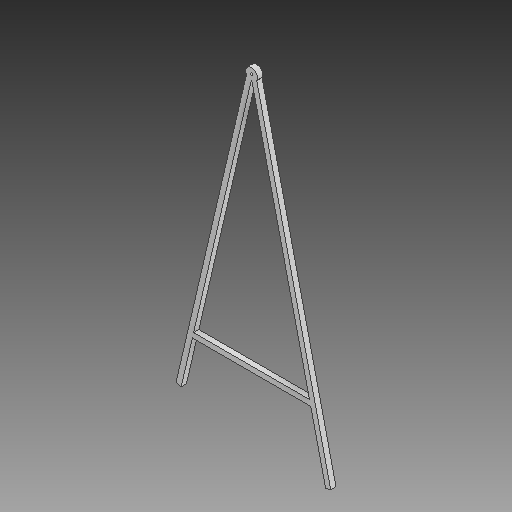
# Autodesk Inventor part: Steher
Saved by Autodesk Inventor 2021 (Build 250183000, 183)
## iProperties
Created: 2021-08-02
Part Number: Steher
Material: Generisch
Document SubType Name: Modeling
Designer: lukas
Density: 1 g/cm^3
Appearance: Vorgabe
Stock Number: Steher
Author: lukas
Autodesk Inventor part; units mm, degrees
ref_plane "YZ Plane" through (0, 0, 0) normal (1, 0, 0) x (0, 1, 0)
ref_plane "XZ Plane" through (0, 0, 0) normal (0, 1, 0) x (-1, 0, 0)
ref_plane "XY Plane" through (0, 0, 0) normal (0, 0, 1) x (1, 0, 0)
sketch "Skizze1" plane through (0, 0, 0) normal (0, 0, 1) x (1, 0, 0)
  line L0 (-523.9247, 0) -> (524.0578, 0) projected
  line L1 (0, -301.1361) -> (0, 1806.8169) projected
  line L2 (350, 0) -> (-350, 0) construction
  line L3 (-350, 0) -> (-374.2129, 6.2512)
  line L4 (-374.2129, 6.2512) -> (-24.346, 1505.6807)
  line L5 (-24.346, 1505.6807) -> (0, 1500)
  line L6 (350, 0) -> (374.346, 5.6807)
  line L7 (374.346, 5.6807) -> (24.346, 1505.6807)
  line L8 (24.346, 1505.6807) -> (0, 1500)
  line L9 (280, 300) -> (-280, 300)
  line L10 (274.1667, 325) -> (-274.1667, 325)
  line L11 (350, 0) -> (280, 300)
  line L12 (274.1667, 325) -> (0, 1500)
  line L13 (-350, 0) -> (-280, 300)
  line L14 (-274.1667, 325) -> (0, 1500)
  point P0 (0, 0)
  point P1 (0, 300)
  dimension "d9" = 700
  dimension "d11" = 300
  dimension "d18" = 1500
  dimension "d19" = 25
  constraints: 26 end point, 4 point on line, 3 parallel, 3 perpendicular, 1 horizontal, 1 symmetric about line
  measures "d9" distance of L2.end L2.start
  measures "d11" distance from line of point (0, 300) L0
  measures "d18" distance from line of L0 L5.end
  measures "d19" distance between parallel lines of L10 L9
extrude "Extrusion2" add sketch "Skizze1" along normal blind 25 contours L3 L4 L5 L14 L10 L1 L9 L13 | L11 L9 L1 L10 L12 L8 L7 L6 | L10 L14 L1 | L1 L12 L10
extrude "Extrusion3" cut sketch "Skizze1" along normal through all contours L10 L14 L1 | L1 L12 L10
sketch "Skizze2" plane through (0, 0, 25) normal (0, 0, 1) x (1, 0, 0)
  circle A0 centre (0, 1520) radius 27.5
  circle A1 centre (0, 1520) radius 5.5
  line L0 (-274.1667, 325) -> (0, 1500) projected
  line L1 (0, 1500) -> (274.1667, 325) projected
  point P0 (0, 0)
  dimension "d38" = 55
  dimension "d39" = 1520
  dimension "d40" = 11
  constraints: 2 centre point, 1 coincident
  measures "d38" diameter of A0
  measures "d39" distance of A0.centre point (0, 0)
  measures "d40" diameter of A1
extrude "Extrusion4" add sketch "Skizze2" against normal blind 25
sketch "Skizze3" plane through (0, 0, 0) normal (0, 0, -1) x (-1, 0, 0)
  line L0 (24.346, 1505.6807) -> (374.2129, 6.2512) projected
  line L1 (350, 0) -> (280, 300) projected
  line L2 (374.2129, 6.2512) -> (350, 0) projected
  line L3 (332.9578, 73.0381) -> (357.3038, 78.7188)
  point P0 (0, 0)
  dimension "d44" = 75
  constraints: 2 end point, 2 point on line, 1 perpendicular
  measures "d44" distance from line of L1.start L3
extrude "Extrusion5" cut sketch "Skizze3" against normal blind 25
